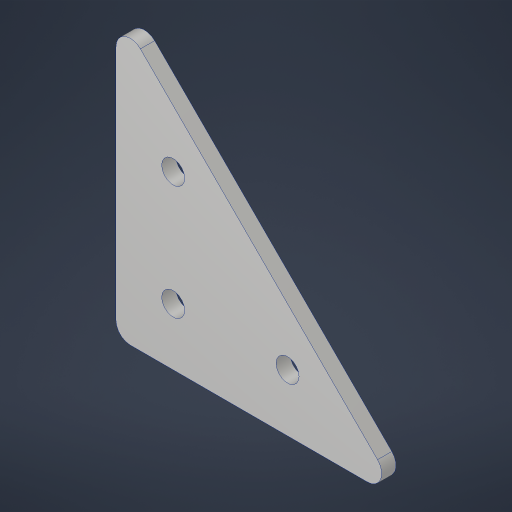
# Autodesk Inventor part: EL2-C-002
Saved by Autodesk Inventor 2023.4 (Build 274418000, 418)
## iProperties
Created: 2025-01-11
Part Number: EL2-C-002
Material: Aluminum 6061
Document SubType Name: Modeling
Designer: brand
Density: 2.7 g/cm^3
Appearance: Aluminum - Flat
Author: brand
Autodesk Inventor part; units mm, degrees
ref_plane "YZ Plane" through (0, 0, 0) normal (1, 0, 0) x (0, 1, 0)
ref_plane "XZ Plane" through (0, 0, 0) normal (0, 1, 0) x (-1, 0, 0)
ref_plane "XY Plane" through (0, 0, 0) normal (0, 0, 1) x (1, 0, 0)
sketch "Sketch1" plane through (0, 0, 0) normal (0, 0, 1) x (1, 0, 0)
  line L0 (0, 0) -> (63.5, 0)
  line L1 (0, 0) -> (0, 63.5)
  line L2 (0, 63.5) -> (63.5, 0)
  dimension "d0" = 63.5
  dimension "d1" = 63.5
  constraints: 6 end point, 1 horizontal, 1 vertical
  measures "d0" distance of L0.start L0.end
  measures "d1" distance of L0.start L1.end
extrude "Extrusion1" add sketch "Sketch1" along normal mid plane 3.175
fillet "Fillet1" radius 3.175 3 edges at (0, 63.5, 0) (63.5, 0, 0) (0, 0, 0)
sketch "Sketch2" plane through (0, 0, 1.5875) normal (0, 0, 1) x (1, 0, 0)
  arc A0 (0, 3.175) -> (3.175, 0) centre (3.175, 3.175) ccw construction
  line L0 (0, 3.175) -> (0, 55.8349) construction
  arc A1 (5.4201, 58.0799) -> (0, 55.8349) centre (3.175, 55.8349) ccw construction
  line L1 (5.4201, 58.0799) -> (58.0799, 5.4201) construction
  arc A2 (55.8349, 0) -> (58.0799, 5.4201) centre (55.8349, 3.175) ccw construction
  line L2 (55.8349, 0) -> (3.175, 0) construction
  point P0 (0, 0)
  point P1 (12.7, 12.7)
  dimension "d5" = 12.7
  dimension "d6" = 12.7
  measures "d5" distance from line of point (12.7, 12.7) L0
  measures "d6" distance from line of L2 point (12.7, 12.7)
hole "Hole1" at (12.7, 12.7, 1.5875) direction (0, 0, -1) diameter 5.1054 end through all clearance for "Flat Head Machine Screw (82)" size "#10" standard "Ansi Unified Screw Threads"
pattern_linear "Rectangular Pattern1" count 2 spacing 25.4 along (1, 0, 0) of "Hole1"
pattern_linear "Rectangular Pattern2" count 2 spacing 25.4 along (0, 1, 0) of "Hole1"
equation "\"d1\" = d0"
body "Solid1"
